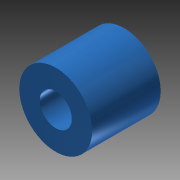
# Autodesk Inventor part: YAxisBearingSpacer
Saved by Autodesk Inventor 2015 SP1 (Build 190203100, 203)
## iProperties
Category: Print
Created: 2014-08-25
Part Number: YAxisBearingSpacer
Material: ABS Plastic
Document SubType Name: Modeling
Designer: t_clevj
Density: 1.06 g/cm^3
Appearance: Cyan
Mass: 0.631065 g
Surface Area: 5.51915 cm^2
Volume: 0.595344 cm^3
Vendor: Jack
Catalog Web Link: N/A
Author: Jack
Title: Y Axis Bearing Spacer
Autodesk Inventor part; units mm, degrees
ref_plane "YZ Plane" through (0, 0, 0) normal (1, 0, 0) x (0, 1, 0)
ref_plane "XZ Plane" through (0, 0, 0) normal (0, 1, 0) x (-1, 0, 0)
ref_plane "XY Plane" through (0, 0, 0) normal (0, 0, 1) x (1, 0, 0)
sketch "Sketch1" plane through (0, 0, 0) normal (0, 1, 0) x (-1, 0, 0)
  circle A0 centre (0, 0) radius 5
  circle A1 centre (0, 0) radius 2.2
  dimension "d0" = 10
  dimension "d1" = 4.4
  constraints: 2 centre point, 2 coincident
  measures "d0" diameter of A0
  measures "d1" diameter of A1
extrude "Extrusion1" add sketch "Sketch1" along normal blind 9.4
body "Solid1"
